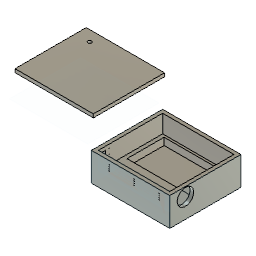
design-3d (Autodesk Fusion 360 design; units mm, degrees)
part number: 2025-10-31-15-14-05-464
Autodesk Fusion 360 part; units mm, degrees
sketch "Sketch1" plane through (0, 0, 0) normal (0, 0, 1) x (1, 0, 0)
  line L0 (50, -50) -> (-60, -50)
  line L1 (-60, -50) -> (-60, 50)
  line L2 (-60, 50) -> (50, 50)
  line L3 (50, 50) -> (50, -50)
  constraint horizontal L0
  constraint vertical L1
  constraint horizontal L2
  constraint vertical L3
extrude "Extrude1" add sketch "Sketch1" along normal blind 30 makes body 1
sketch "Sketch2" plane through (0, 0, 30) normal (0, 0, 1) x (-1, 0, 0)
  line L0 (-50, -50) -> (60, -50)
  line L1 (60, -50) -> (60, 50)
  line L2 (60, 50) -> (-50, 50)
  line L3 (-50, 50) -> (-50, -50)
  line L4 (-45, 45) -> (55, 45)
  line L5 (55, 45) -> (55, -45)
  line L6 (55, -45) -> (-45, -45)
  line L7 (-45, -45) -> (-45, 45)
  constraint horizontal L4
  constraint vertical L5
  constraint horizontal L6
  constraint vertical L7
extrude "Extrude2" cut sketch "Sketch2" against normal blind 25 contours L4 L5 L6 L7 bodies 1
sketch "Sketch3" plane through (0, 0, 5) normal (0, 0, 1) x (-1, 0, 0)
  line L0 (-45, -45) -> (55, -45)
  line L1 (55, -45) -> (55, 45)
  line L2 (55, 45) -> (-45, 45)
  line L3 (-45, 45) -> (-45, -45)
  line L4 (-40.1539, 10.0968) -> (49.8457, 10.0968)
  line L5 (49.8457, 10.0968) -> (49.8457, -41.9032)
  line L6 (49.8457, -41.9032) -> (-40.1539, -41.9032)
  line L7 (-40.1539, -41.9032) -> (-40.1539, 10.0968)
  dimension "d5" = 52
  constraint horizontal L4
  constraint vertical L5
  constraint horizontal L6
  constraint vertical L7
  measures "d5" distance of L4.start L6.end
extrude "Extrude3" add 1 faces at (13.3333, -16.6667, 0) along direction (0, 0, -1) blind 10 on bodies 1 bodies 1
extrude "Extrude4" cut sketch "Sketch3" against normal blind 10 contours L4 L5 L6 L7 bodies 1
sketch "Sketch4" plane through (0, -50, 0) normal (0, -1, 0) x (1, 0, 0)
  line L0 (50, -10) -> (50, 30)
  line L1 (50, 30) -> (-60, 30)
  line L2 (-60, 30) -> (-60, -10)
  line L3 (-60, -10) -> (50, -10)
sketch "Sketch5" plane through (0, -45, 0) normal (0, 1, 0) x (-1, 0, 0)
  line L0 (55, 30) -> (-45, 30)
  line L1 (-45, 30) -> (-45, 5)
  line L2 (-45, 5) -> (55, 5)
  line L3 (55, 5) -> (55, 30)
sketch "Sketch6" plane through (0, -45, 0) normal (0, 1, 0) x (-1, 0, 0)
sketch "Sketch7" plane through (0, -50, 0) normal (0, -1, 0) x (1, 0, 0)
sketch "Sketch8" plane through (0, -50, 0) normal (0, -1, 0) x (1, 0, 0)
sketch "Sketch9" plane through (0, -50, 0) normal (0, -1, 0) x (1, 0, 0)
  circle A0 centre (-35, 25) radius 0.5
  point P0 (0, 25)
  point P1 (35, 25)
  point P2 (0, 22.46)
  point P3 (35, 22.46)
  point P4 (-35, 22.46)
  point P5 (35, 17.38)
  point P6 (-35, 17.38)
  point P7 (0, 19.92)
  point P8 (35, 19.92)
  point P9 (-35, 19.92)
  point P10 (0, 17.38)
  dimension "d12" = 1
  measures "d12" diameter of A0
extrude "Extrude5" cut sketch "Sketch9" against normal blind 28 bodies 1
sketch "Sketch10" plane through (0, -50, 0) normal (0, -1, 0) x (1, 0, 0)
  circle A0 centre (0, 25) radius 0.5
  dimension "d15" = 1
  measures "d15" diameter of A0
extrude "Extrude6" cut sketch "Sketch10" against normal blind 30 bodies 1
sketch "Sketch11" plane through (0, -50, 0) normal (0, -1, 0) x (1, 0, 0)
  circle A0 centre (35, 25) radius 0.5
  dimension "d18" = 1
  measures "d18" diameter of A0
extrude "Extrude7" cut sketch "Sketch11" against normal blind 30 bodies 1
sketch "Sketch12" plane through (0, -50, 0) normal (0, -1, 0) x (1, 0, 0)
  circle A0 centre (-35, 22.46) radius 0.5
  dimension "d21" = 1
  measures "d21" diameter of A0
extrude "Extrude8" cut sketch "Sketch12" against normal blind 36 bodies 1
sketch "Sketch13" plane through (0, -50, 0) normal (0, -1, 0) x (1, 0, 0)
  circle A0 centre (0, 22.46) radius 0.5
  dimension "d24" = 1
  measures "d24" diameter of A0
extrude "Extrude9" cut sketch "Sketch13" against normal blind 36 bodies 1
sketch "Sketch14" plane through (0, -50, 0) normal (0, -1, 0) x (1, 0, 0)
  circle A0 centre (35, 22.46) radius 0.5
  dimension "d27" = 1
  measures "d27" diameter of A0
extrude "Extrude10" cut sketch "Sketch14" against normal blind 51 bodies 1
sketch "Sketch15" plane through (0, -50, 0) normal (0, -1, 0) x (1, 0, 0)
  circle A0 centre (-35, 19.92) radius 0.5
  dimension "d30" = 1
  measures "d30" diameter of A0
extrude "Extrude11" cut sketch "Sketch15" against normal blind 45 bodies 1
sketch "Sketch16" plane through (0, -45, 0) normal (0, 1, 0) x (-1, 0, 0)
sketch "Sketch17" plane through (0, -50, 0) normal (0, -1, 0) x (1, 0, 0)
  circle A0 centre (0, 19.92) radius 0.5
  dimension "d33" = 1
  measures "d33" diameter of A0
extrude "Extrude12" cut sketch "Sketch17" against normal blind 53 bodies 1
sketch "Sketch18" plane through (0, -50, 0) normal (0, -1, 0) x (1, 0, 0)
  circle A0 centre (35, 19.92) radius 0.5
  dimension "d36" = 1
  measures "d36" diameter of A0
extrude "Extrude13" cut sketch "Sketch18" against normal blind 34 bodies 1
sketch "Sketch19" plane through (0, -50, 0) normal (0, -1, 0) x (1, 0, 0)
  circle A0 centre (-35, 17.38) radius 0.5
  dimension "d39" = 1
  measures "d39" diameter of A0
sketch "Sketch20" plane through (0, -50, 0) normal (0, -1, 0) x (1, 0, 0)
extrude "Extrude14" cut sketch "Sketch19" against normal blind 60 bodies 1
sketch "Sketch21" plane through (0, -50, 0) normal (0, -1, 0) x (1, 0, 0)
  circle A0 centre (0, 17.38) radius 0.5
  dimension "d42" = 1
  measures "d42" diameter of A0
extrude "Extrude15" cut sketch "Sketch21" against normal blind 59 bodies 1
sketch "Sketch22" plane through (0, -50, 0) normal (0, -1, 0) x (1, 0, 0)
  circle A0 centre (35, 17.38) radius 0.5
  dimension "d45" = 1
  measures "d45" diameter of A0
extrude "Extrude16" cut sketch "Sketch22" against normal blind 50 bodies 1
sketch "Sketch23" plane through (50, 0, 0) normal (1, 0, 0) x (0, 1, 0)
  line L0 (50, -10) -> (50, 30)
  line L1 (50, 30) -> (-50, 30)
  line L2 (-50, 30) -> (-50, -10)
  line L3 (-50, -10) -> (50, -10)
sketch "Sketch24" plane through (50, 0, 0) normal (1, 0, 0) x (0, 1, 0)
sketch "Sketch25" plane through (50, 0, 0) normal (1, 0, 0) x (0, 1, 0)
sketch "Sketch26" plane through (0, 0, 0) normal (1, 0, 0) x (0, 1, 0)
sketch "Sketch27" plane through (50, 0, 0) normal (1, 0, 0) x (0, 1, 0)
  circle A0 centre (-28, 17.5) radius 11.5
  dimension "d48" = 23
  measures "d48" diameter of A0
extrude "Extrude17" cut sketch "Sketch27" against normal blind 40 bodies 1
sketch "Sketch28" plane through (-60, 0, 0) normal (-1, 0, 0) x (0, -1, 0)
  line L0 (50, -10) -> (50, 30)
  line L1 (50, 30) -> (-50, 30)
  line L2 (-50, 30) -> (-50, -10)
  line L3 (-50, -10) -> (50, -10)
  line L4 (35, 25) -> (40, 25)
  line L5 (40, 25) -> (40, 15)
  line L6 (40, 15) -> (35, 15)
  line L7 (35, 15) -> (35, 25)
  constraint horizontal L4
  constraint vertical L5
  constraint horizontal L6
  constraint vertical L7
extrude "Extrude18" cut sketch "Sketch28" against normal blind 30 contours L4 L5 L6 L7 bodies 1
sketch "Sketch29" plane through (0, 0, 30) normal (0, 0, 1) x (-1, 0, 0)
  line L0 (55, 45) -> (55, -45)
  line L1 (55, -45) -> (-45, -45)
  line L2 (-45, -45) -> (-45, 45)
  line L3 (-45, 45) -> (55, 45)
  line L4 (-50, -50) -> (60, -50)
  line L5 (60, -50) -> (60, 50)
  line L6 (60, 50) -> (-50, 50)
  line L7 (-50, 50) -> (-50, -50)
  line L8 (174.9797, 50) -> (64.9797, 50)
  line L9 (64.9797, 50) -> (64.9797, -50)
  line L10 (64.9797, -50) -> (174.9797, -50)
  line L11 (174.9797, -50) -> (174.9797, 50)
  constraint horizontal L8
  constraint vertical L9
  constraint horizontal L10
  constraint vertical L11
  constraint coincident L4 L9.end
extrude "Extrude19" add sketch "Sketch29" along normal blind 5 separate body contours L8 L9 L10 L11 makes body 2
sketch "Sketch30" plane through (0, 0, 35) normal (0, 0, 1) x (-1, 0, 0)
  line L0 (174.9797, -50) -> (174.9797, 50)
  line L1 (174.9797, 50) -> (64.9797, 50)
  line L2 (64.9797, 50) -> (64.9797, -50)
  line L3 (64.9797, -50) -> (174.9797, -50)
sketch "Sketch31" plane through (0, 0, 35) normal (0, 0, 1) x (-1, 0, 0)
  circle A0 centre (155, -35) radius 2.5
  dimension "d56" = 5
  measures "d56" diameter of A0
extrude "Extrude20" cut sketch "Sketch31" against normal blind 20 bodies 2
move_body "Move1" bodies 2 to x (1, 0, 0) y (0, 1, 0) z (0, 0, 1) at (0, 7.8419, 32.8123)
sketch "Sketch32" plane through (-60, 0, 0) normal (-1, 0, 0) x (0, -1, 0)
  line L0 (40, 25) -> (40, 15)
  line L1 (40, 15) -> (35, 15)
  line L2 (35, 15) -> (35, 25)
  line L3 (35, 25) -> (40, 25)
  line L4 (50, -10) -> (50, 30)
  line L5 (50, 30) -> (-50, 30)
  line L6 (-50, 30) -> (-50, -10)
  line L7 (-50, -10) -> (50, -10)
  circle A0 centre (30, 25) radius 0.5
  dimension "d59" = 1
  measures "d59" diameter of A0
extrude "Extrude21" cut sketch "Sketch32" against normal blind 25 contours A0 bodies 1
sketch "Sketch33" plane through (-60, 0, 0) normal (-1, 0, 0) x (0, -1, 0)
  circle A0 centre (30, 25) radius 0.5
  line L0 (40, 25) -> (40, 15)
  line L1 (40, 15) -> (35, 15)
  line L2 (35, 15) -> (35, 25)
  line L3 (35, 25) -> (40, 25)
  line L4 (50, -10) -> (50, 30)
  line L5 (50, 30) -> (-50, 30)
  line L6 (-50, 30) -> (-50, -10)
  line L7 (-50, -10) -> (50, -10)
sketch "Sketch34" plane through (-60, 0, 0) normal (-1, 0, 0) x (0, -1, 0)
sketch "Sketch35" plane through (-60, 0, 0) normal (-1, 0, 0) x (0, -1, 0)
  circle A0 centre (30, 17.5) radius 0.5
  dimension "d64" = 1
  measures "d64" diameter of A0
extrude "Extrude22" cut sketch "Sketch35" against normal blind 135 bodies 1
